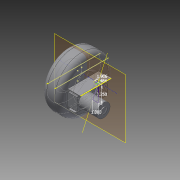
# Autodesk Inventor part: Snow Tire Wheel with Gearbox and CIM
Saved by Autodesk Inventor 2015 (Build 190159000, 159)
## iProperties
Created: 2016-01-18
Part Number: Snow Tire Wheel with Gearbox and CIM
Material: Generic
Document SubType Name: Modeling
Designer: sethbattis
Density: 1 g/cm^3
Appearance: Default
Author: sethbattis
Autodesk Inventor part; units mm, degrees
ref_plane "YZ Plane" through (0, 0, 0) normal (1, 0, 0) x (0, 1, 0)
ref_plane "XZ Plane" through (0, 0, 0) normal (0, 1, 0) x (-1, 0, 0)
ref_plane "XY Plane" through (0, 0, 0) normal (0, 0, 1) x (1, 0, 0)
sketch "Sketch1" plane through (0, 0, 0) normal (0, 0, 1) x (1, 0, 0)
  line L0 (-44.45, 127) -> (44.45, 127)
  line L1 (44.45, 127) -> (44.45, 50.8)
  line L2 (-44.45, 50.8) -> (-44.45, 127)
  line L3 (31.75, 50.8) -> (31.75, 0)
  line L4 (31.75, 0) -> (-31.75, 0)
  line L5 (-31.75, 0) -> (-31.75, 50.8)
  line L6 (-44.45, 50.8) -> (-31.75, 50.8)
  line L7 (31.75, 50.8) -> (44.45, 50.8)
  line L8 (152.4, 0) -> (-152.4, 0) construction
  point P0 (0, 0)
  dimension "d0" = 88.9
  dimension "d1" = 76.2
  dimension "d3" = 44.45
  dimension "d4" = 63.5
  dimension "d12" = 152.4
  dimension "d13" = 152.4
  constraints: 18 end point, 3 horizontal, 2 parallel, 1 collinear, 1 perpendicular
  measures "d0" distance of L1.end L2.start
  measures "d1" distance of L0.end L1.end
  measures "d3" distance from line of point (0, 0) L2
  measures "d4" distance of L3.end L4.end
  measures "d12" distance of point (0, 0) L8.end
  measures "d13" distance of L8.start point (0, 0)
revolve "Snow Blower Tire" add sketch "Sketch1" angle 360 about axis through (31.75, 0, 0) along (-1, 0, 0)
fillet "Fillet1" radius 25.4 2 edges at (44.45, -127, 0) (-44.45, -127, 0)
chamfer "Chamfer1" distance 12.7 angle 45 2 edges at (44.45, -50.8, 0) (-44.45, -50.8, 0)
sketch "Sketch2" plane through (0, 0, 0) normal (0, 0, 1) x (1, 0, 0)
  line L0 (50.8, 42.0687) -> (50.8, -42.0688)
  line L1 (50.8, -42.0688) -> (85.725, -42.0688)
  line L2 (85.725, -42.0688) -> (85.725, -38.8938)
  line L3 (85.725, -38.8938) -> (53.975, -38.8938)
  line L4 (53.975, -38.8938) -> (53.975, -31.75)
  line L5 (53.975, 38.8937) -> (109.3812, 38.8938)
  line L6 (109.3812, 38.8938) -> (109.3812, 42.0688)
  line L7 (109.3812, 42.0688) -> (50.8, 42.0687)
  line L8 (-86.9955, 0) -> (165.7829, 0) construction
  line L9 (0, -177.8) -> (0, 177.8) projected
  line L10 (53.975, 31.75) -> (95.25, 31.75)
  line L11 (95.25, 31.75) -> (95.25, -31.75)
  line L12 (95.25, -31.75) -> (53.975, -31.75)
  line L13 (53.975, 31.75) -> (53.975, 38.8937)
  line L14 (53.975, 38.8937) -> (50.8, 38.8937) construction
  point P0 (0, 0)
  dimension "d14" = 84.1375
  dimension "d15" = 34.925
  dimension "d16" = 3.175
  dimension "d19" = 42.0688
  dimension "d23" = 50.8
  dimension "d28" = 41.275
  dimension "d29" = 63.5
  constraints: 28 end point, 9 perpendicular, 3 equal length, 3 horizontal, 2 parallel, 1 point on line, 1 vertical
  measures "d14" distance of L0.start L0.end
  measures "d15" distance of L0.end L1.end
  measures "d16" distance of L1.end L2.end
  measures "d19" distance between parallel lines of L8 L7
  measures "d23" distance between parallel lines of L0 L9
  measures "d28" distance of L11.end L4.end
  measures "d29" distance of L10.end L11.end
extrude "Gearbox" add sketch "Sketch2" along normal blind 96.8375 and the other way blind 48.4124
sketch "Sketch6" plane through (95.25, -31.75, 96.8375) normal (1, 0, 0) x (0, 0, -1)
  line L0 (0, 0) -> (0, 63.5) projected
  line L1 (145.2499, 63.5) -> (0, 63.5) projected
  line L2 (145.2499, 0) -> (0, 0) projected
  line L3 (145.2499, 63.5) -> (145.2499, 0) projected
  line L4 (0, 31.75) -> (145.2499, 31.75) construction
  line L5 (38.1, 63.5) -> (38.1, 0) construction
  circle A0 centre (38.1, 31.75) radius 31.75
  point P0 (96.8375, 31.75)
  dimension "d40" = 38.1
  dimension "d41" = 63.5
  constraints: 4 end point, 3 midpoint, 2 point on line, 1 centre point, 1 perpendicular
  measures "d40" distance between parallel lines of L5 L0
  measures "d41" diameter of A0
extrude "CIM" add sketch "Sketch6" along normal blind 85.344 contours A0
sketch "Sketch7" plane through (180.594, 0, 58.7375) normal (1, 0, 0) x (0, 0, -1)
  circle A0 centre (0, 0) radius 14.2875
  point P0 (58.7375, 0)
  dimension "d44" = 28.575
  constraints: 1 centre point
  measures "d44" diameter of A0
extrude "Extrusion6" add sketch "Sketch7" along normal blind 4.7625
sketch "Sketch8" plane through (50.8, 42.0688, 96.8375) normal (0, 1, 0) x (1, 0, 0)
  line L0 (-31.75, -30.1625) -> (-31.75, 223.8375) projected
  line L1 (-31.75, -30.1625) -> (-31.75, 223.8375) projected
  line L2 (-69.85, 223.8375) -> (-69.85, -30.1625) projected
  line L3 (-144.3028, 96.8375) -> (140.0403, 96.8375) construction
  line L4 (58.5812, 145.2499) -> (58.5812, 0) projected
  line L5 (46.2781, 104.5566) -> (46.2781, 86.4461) construction
  point P0 (-50.8, 96.8375)
  point P1 (46.2781, 96.8375)
  point P2 (46.2781, 96.8375)
  dimension "d69" = 12.3031
  dimension "d70" = 48.4124
  constraints: 4 end point, 2 horizontal, 1 coincident, 1 vertical
  measures "d69" distance from line of L4 point (46.278, 96.838)
  measures "d70" vertical distance of L4.start point (46.278, 96.838)
fillet "Fillet3" radius 3.175 8 edges at (109.3812, 40.4813, 96.8375) (109.3812, 40.4813, -48.4124) (85.725, -40.4813, 96.8375) (85.725, -40.4813, -48.4124) (74.6125, 31.75, 96.8375) (74.6125, -31.75, 96.8375) (74.6125, -31.75, -48.4124) (74.6125, 31.75, -48.4124)
ref_plane "Work Plane6" through (-93.5028, 42.0687, 0) normal (0, 0, 1) x (1, 0, 0)
sketch "Sketch16" plane through (-93.5028, 42.0687, 0) normal (0, 0, 1) x (1, 0, 0)
  line L0 (190.5809, 0) -> (165.1809, -82.55)
  line L1 (165.1809, -82.55) -> (190.5809, -82.55)
  line L2 (190.5809, -82.55) -> (190.5809, 0)
  point P0 (93.5028, -42.0688)
  dimension "d71" = 82.55
  dimension "d72" = 25.4
  constraints: 6 end point, 1 horizontal, 1 vertical
  measures "d71" distance of L1.end L0.start
  measures "d72" distance of L0.end L1.end
ref_plane "Work Plane7" through (97.0781, 42.0688, 0) normal (-0.2940858, -0.955779, 0) x (0.955779, -0.2940858, 0)
sketch "Sketch17" plane through (97.0781, 42.0688, 0) normal (-0.2940858, -0.955779, 0) x (0.955779, -0.2940858, 0)
  line L0 (0, 0) -> (0, -10.9395)
  line L1 (0, 0) -> (0, 10.9068)
  point P0 (-80.4134, 0)
  constraints: 4 end point, 2 vertical
equation "\"d19\" = 0.5 * d14"
body "Solid1"
